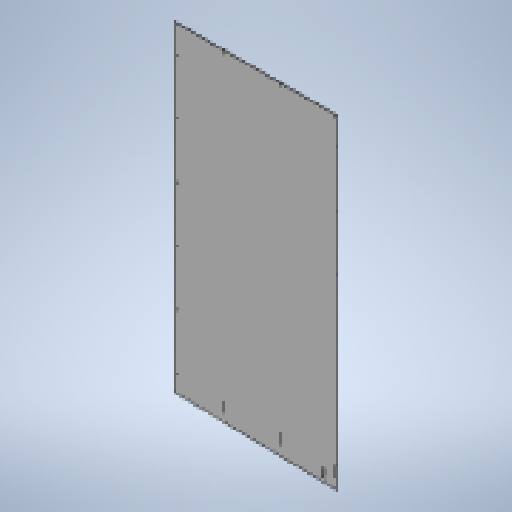
# Autodesk Inventor part: GBK 2211 shield 4
Saved by Autodesk Inventor 2026.2 (Build 302298010, 298A)
## iProperties
Created: 2026-04-17
Part Number: GBK 2211 shield 4
Material: Steel
Document SubType Name: Sheet Metal
Designer: pokla
Stock Number: 2214
Mass: 138487 g
Surface Area: 88564.8 cm^2
Volume: 17641.6 cm^3
Density: 7.85 g/cm^3
Flat Pattern Width: 148 cm
Flat Pattern Length: 292 cm
Flat Pattern Area: 43216 cm^2
Sheet Metal Rule: Default_mm
Sheet Metal Width: 1480,000 mm
Sheet Metal Length: 2920,000 mm
Sheet Metal Area: 4321600,000 mm^2
Appearance: Default
Author: admin
Autodesk Inventor part; units mm, degrees
ref_plane "YZ Plane" through (0, 0, 0) normal (1, 0, 0) x (0, 1, 0)
ref_plane "XZ Plane" through (0, 0, 0) normal (0, 1, 0) x (-1, 0, 0)
ref_plane "XY Plane" through (0, 0, 0) normal (0, 0, 1) x (1, 0, 0)
sketch "Sketch1" plane through (0, 0, 0) normal (0, 0, 1) x (1, 0, 0)
  line L0 (740, -1490) -> (-740, -1490)
  line L1 (-740, -1490) -> (-740, 1490)
  line L2 (-740, 1490) -> (740, 1490)
  line L3 (740, 1490) -> (740, -1490)
  line L4 (740, -1490) -> (-740, 1490) construction
  line L5 (-740, -1490) -> (740, 1490) construction
  line L6 (740, -1430) -> (-740, -1396.4141)
  point P0 (0, 0)
  dimension "d0" = 1480
  dimension "d1" = 2980
  dimension "d3" = 1.3
  dimension "d4" = 60
  measures "d0" distance of L1.end L2.end
  measures "d1" distance of L0.end L1.end
  measures "d3" angle of L0 L6
  measures "d4" distance of L0.start L6.start
extrude "Plate1" add sketch "Sketch1" along normal blind 4 contours L6 L1 L2 L3
sketch "Sketch2" plane through (0, 0, 4) normal (0, 0, 1) x (1, 0, 0)
  line L0 (621.6658, -1316.5027) -> (621.6658, -1674.1932) construction
  line L1 (621.6658, -1674.1932) -> (530.4095, -1674.1932) construction
  line L2 (530.4095, -1674.1932) -> (530.4095, -1316.5027) construction
  line L3 (530.4095, -1316.5027) -> (621.6658, -1316.5027) construction
  line L4 (789.9949, -1235.5) -> (729.9949, -1235.5) projected
  line L5 (729.9949, -1239.5) -> (729.9949, -1235.5) projected
  line L6 (710.2434, -1243) -> (710.2434, -1340) projected
  line L7 (710.2434, -1340) -> (706.2444, -1340) projected
  ellipse E0 centre (710.2434, 1484.5) end of major axis (710.2434, 1514.5) minor radius 0.6803 (710.2434, 1454.5) -> (710.2434, 1514.5) ccw projected
  line L8 (710.2434, 1454.5) -> (706.2444, 1454.5) projected
  line L9 (789.9949, 1247.8333) -> (729.9949, 1247.8333) projected
  line L10 (729.9949, 1243.8333) -> (729.9949, 1247.8333) projected
  line L11 (789.9949, 751.1667) -> (729.9949, 751.1667) projected
  line L12 (729.9949, 747.1667) -> (729.9949, 751.1667) projected
  line L13 (789.9949, 254.5) -> (729.9949, 254.5) projected
  line L14 (729.9949, 250.5) -> (729.9949, 254.5) projected
  line L15 (789.9949, -242.1667) -> (729.9949, -242.1667) projected
  line L16 (729.9949, -246.1667) -> (729.9949, -242.1667) projected
  line L17 (789.9949, -738.8333) -> (729.9949, -738.8333) projected
  line L18 (729.9949, -742.8333) -> (729.9949, -738.8333) projected
  ellipse E1 centre (210.1148, 1484.5) end of major axis (210.1148, 1514.5) minor radius 0.6803 (210.1148, 1454.5) -> (210.1148, 1514.5) ccw projected
  line L19 (210.1148, 1454.5) -> (206.1159, 1454.5) projected
  ellipse E2 centre (-290.0138, 1484.5) end of major axis (-290.0138, 1514.5) minor radius 0.6803 (-290.0138, 1454.5) -> (-290.0138, 1514.5) ccw projected
  line L20 (-290.0138, 1454.5) -> (-294.0127, 1454.5) projected
  line L21 (-690.0051, 1247.8333) -> (-719.3249, 1247.8333) projected
  line L22 (-690.0051, 1243.8333) -> (-690.0051, 1247.8333) projected
  line L23 (-690.0051, 751.1667) -> (-719.3249, 751.1667) projected
  line L24 (-690.0051, 747.1667) -> (-690.0051, 751.1667) projected
  line L25 (-690.0051, 254.5) -> (-719.3249, 254.5) projected
  line L26 (-690.0051, 250.5) -> (-690.0051, 254.5) projected
  line L27 (-690.0051, -242.1667) -> (-719.3249, -242.1667) projected
  line L28 (-690.0051, -246.1667) -> (-690.0051, -242.1667) projected
  line L29 (-690.0051, -738.8333) -> (-719.3249, -738.8333) projected
  line L30 (-690.0051, -742.8333) -> (-690.0051, -738.8333) projected
  line L31 (-690.0051, -1235.5) -> (-719.3249, -1235.5) projected
  line L32 (-690.0051, -1239.5) -> (-690.0051, -1235.5) projected
  line L33 (-290.0138, -1243) -> (-290.0138, -1340) projected
  line L34 (-290.0138, -1340) -> (-294.0127, -1340) projected
  line L35 (210.1148, -1243) -> (210.1148, -1340) projected
  line L36 (210.1148, -1340) -> (206.1159, -1340) projected
  point P0 (0, 0)
  constraints: 5 other
mark "Mark1"
equation "\"d0\" = Лист_ширина"
equation "\"d2\" = Thickness"
equation "\"BendRadius\" = Thickness"
equation "\"BendReliefWidth\" = Thickness"
equation "\"BendReliefDepth\" = 0.5 * Thickness"
equation "\"CornerReliefSize\" = 4 * Thickness"
equation "\"MinimumRemnant\" = 2 * Thickness"
equation "\"TransitionRadius\" = BendRadius"
equation "\"JacobiRadiusSize\" = BendRadius"
equation "\"GapSize\" = Thickness"
equation "\"Лист_ширина\" = 1480"
equation "\"Thickness\" = 4"
body "Solid1"
